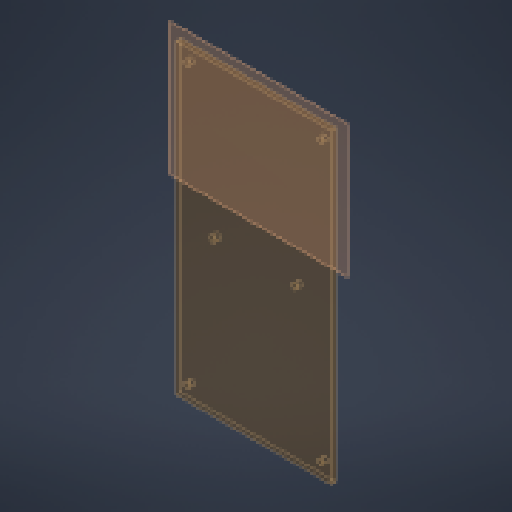
# Autodesk Inventor part: BP_CoverPlateAcrylic
Saved by Autodesk Inventor 2026.1 (Build 301233020, 233B)
## iProperties
Created: 2025-09-13
Part Number: BP_CoverPlateAcrylic
Material: PMMA Plastic
Document SubType Name: Modeling
Designer: atrus
Density: 1.188 g/cm^3
Appearance: Polycarbonate - Smoked
Author: atrus
Autodesk Inventor part; units mm, degrees
ref_plane "YZ Plane" through (0, 0, 0) normal (1, 0, 0) x (0, 1, 0)
ref_plane "XZ Plane" through (0, 0, 0) normal (0, 1, 0) x (-1, 0, 0)
ref_plane "XY Plane" through (0, 0, 0) normal (0, 0, 1) x (1, 0, 0)
ref_plane "Work Plane1" through (0, 0, 0) normal (0, 0, 1) x (1, 0, 0)
sketch "Sketch1" plane through (0, 0, 0) normal (0, 0, 1) x (1, 0, 0)
  line L0 (-10.216, 5.2) -> (85.116, 5.2)
  line L1 (85.116, 5.2) -> (85.116, -183)
  line L2 (85.116, -183) -> (-10.216, -183)
  line L3 (-10.216, -183) -> (-10.216, 5.2)
  line L4 (0, 0.2) -> (74.9, 0.2) construction
  line L5 (0, 0.2) -> (0, -6.8) projected
  line L6 (-8.95, -53) -> (-8.95, -6.8) projected
  line L7 (-8.95, -6.8) -> (0, -6.8) projected
  line L8 (-10.416, 5.4) -> (85.316, 5.4) projected
  circle A0 centre (-3.5, -3.3) radius 1.9 projected
  circle A1 centre (78.4, -3.3) radius 1.9 projected
  line L9 (-10.416, 5.4) -> (-10.416, -67) projected
  line L10 (-10.416, -67) -> (0, -67) projected
  line L11 (0, -53) -> (0, -67) projected
  line L12 (0, -53) -> (-8.95, -53) projected
  line L13 (-8.95, -53) -> (-8.95, -6.8) projected
  line L14 (-8.95, -6.8) -> (0, -6.8) projected
  line L15 (0, 0.2) -> (0, -6.8) projected
  line L16 (0, 0.2) -> (74.9, 0.2) projected
  line L17 (74.9, -6.8) -> (74.9, 0.2) projected
  line L18 (74.9, -6.8) -> (83.85, -6.8) projected
  line L19 (83.85, -6.8) -> (83.85, -53) projected
  line L20 (83.85, -53) -> (74.9, -53) projected
  line L21 (74.9, -67) -> (74.9, -53) projected
  line L22 (74.9, -67) -> (85.316, -67) projected
  line L23 (85.316, -67) -> (85.316, 5.4) projected
  line L24 (85.316, 5.4) -> (-10.416, 5.4) projected
  circle A2 centre (78.4, -174.4) radius 1.9 projected
  circle A3 centre (-3.5, -174.4) radius 1.9 projected
  line L25 (85.316, -183.2) -> (85.316, -110.8) projected
  line L26 (85.316, -110.8) -> (74.9, -110.8) projected
  line L27 (74.9, -110.8) -> (74.9, -124.8) projected
  line L28 (74.9, -124.8) -> (83.85, -124.8) projected
  line L29 (83.85, -124.8) -> (83.85, -170.9) projected
  line L30 (83.85, -170.9) -> (74.9, -170.9) projected
  line L31 (74.9, -170.9) -> (74.9, -177.9) projected
  line L32 (0, -177.9) -> (74.9, -177.9) projected
  line L33 (0, -170.9) -> (0, -177.9) projected
  line L34 (0, -170.9) -> (-8.95, -170.9) projected
  line L35 (-8.95, -170.9) -> (-8.95, -124.8) projected
  line L36 (-8.95, -124.8) -> (0, -124.8) projected
  line L37 (0, -110.8) -> (0, -124.8) projected
  line L38 (0, -110.8) -> (-10.416, -110.8) projected
  line L39 (-10.416, -110.8) -> (-10.416, -183.2) projected
  line L40 (-10.416, -183.2) -> (85.316, -183.2) projected
  circle A4 centre (78.4, -174.4) radius 1.9 projected
  circle A5 centre (-3.5, -174.4) radius 1.9 projected
  line L41 (85.316, -183.2) -> (85.316, -110.8) projected
  line L42 (85.316, -110.8) -> (74.9, -110.8) projected
  line L43 (74.9, -110.8) -> (74.9, -124.8) projected
  line L44 (74.9, -124.8) -> (83.85, -124.8) projected
  line L45 (83.85, -124.8) -> (83.85, -170.9) projected
  line L46 (83.85, -170.9) -> (74.9, -170.9) projected
  line L47 (74.9, -170.9) -> (74.9, -177.9) projected
  line L48 (0, -177.9) -> (74.9, -177.9) projected
  line L49 (0, -170.9) -> (0, -177.9) projected
  line L50 (0, -170.9) -> (-8.95, -170.9) projected
  line L51 (-8.95, -170.9) -> (-8.95, -124.8) projected
  line L52 (-8.95, -124.8) -> (0, -124.8) projected
  line L53 (0, -110.8) -> (0, -124.8) projected
  line L54 (0, -110.8) -> (-10.416, -110.8) projected
  line L55 (-10.416, -110.8) -> (-10.416, -183.2) projected
  line L56 (-10.416, -183.2) -> (85.316, -183.2) projected
  point P0 (0, 0)
  dimension "d9" = 0.2
  dimension "d12" = 0.2
  dimension "d13" = 0.2
  dimension "d14" = 0.2
  constraints: 8 end point, 2 parallel, 1 horizontal, 1 perpendicular
  measures "d9" distance between parallel lines of L8 L0
  measures "d12" distance between parallel lines of L40 L2
  measures "d13" distance between parallel lines of L39 L3
  measures "d14" distance between parallel lines of L23 L1
extrude "Extrusion1" add sketch "Sketch1" along normal blind 3 contours L0 L1 L22 L21 L20 L19 L18 L17 L16 L5 L7 L6 L12 L11 L10 L3 | L10 L11 L12 L6 L7 L5 L16 L17 L18 L19 L20 L21 L22 L1 L26 L27 L28 L29 L30 L31 L32 L33 L34 L35 L36 L37 L38 L3 | L38 L37 L36 L35 L34 L33 L32 L31 L30 L29 L28 L27 L26 L1 L2 L3 | A0 | A1 | A2 | A3
sketch "Sketch2" plane through (0, 0, 3) normal (0, 0, 1) x (1, 0, 0)
  circle A0 centre (78.4, -3.3) radius 1.9 projected
  circle A1 centre (-3.5, -3.3) radius 1.9 projected
  circle A2 centre (12.45, -88.9) radius 1.9 projected
  circle A3 centre (62.45, -88.9) radius 1.9 projected
  circle A4 centre (78.4, -174.4) radius 1.9 projected
  circle A5 centre (-3.5, -174.4) radius 1.9 projected
  point P0 (0, 0)
extrude "Extrusion2" cut sketch "Sketch2" against normal blind 3
body "Solid1"
